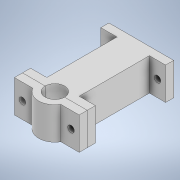
# Autodesk Inventor part: Держатель лазера
Saved by Autodesk Inventor 2022 (Build 260153000, 153)
## iProperties
Created: 2022-06-19
Part Number: Держатель лазера
Material: Типовые
Document SubType Name: Modeling
Designer: Admin
Density: 1 g/cm^3
Appearance: По умолчанию
Author: Admin
Autodesk Inventor part; units mm, degrees
ref_plane "YZ Plane" through (0, 0, 0) normal (1, 0, 0) x (0, 1, 0)
ref_plane "XZ Plane" through (0, 0, 0) normal (0, 1, 0) x (-1, 0, 0)
ref_plane "XY Plane" through (0, 0, 0) normal (0, 0, 1) x (1, 0, 0)
sketch "Эскиз1" plane through (0, 0, 0) normal (0, 0, 1) x (1, 0, 0)
  line L0 (20, -10) -> (-20, -10)
  line L1 (-20, -10) -> (-20, 10)
  line L2 (-20, 10) -> (20, 10)
  line L3 (20, 10) -> (20, -10)
  line L4 (20, -10) -> (-20, 10) construction
  line L5 (-20, -10) -> (20, 10) construction
  circle A0 centre (-15, 0) radius 2
  circle A1 centre (15, 0) radius 2
  line L6 (-10, -10) -> (10, -10)
  line L7 (10, -10) -> (10, 10)
  line L8 (10, 10) -> (-10, 10)
  line L9 (-10, 10) -> (-10, -10)
  line L10 (-10, -10) -> (10, 10) construction
  line L11 (10, -10) -> (-10, 10) construction
  point P0 (0, 0)
  point P1 (0, 0)
  dimension "d0" = 40
  dimension "d1" = 20
  dimension "d2" = 4
  dimension "d3" = 4
  dimension "d4" = 15
  dimension "d5" = 15
  dimension "d6" = 20
  constraints: 24 end point, 5 midpoint, 4 parallel, 2 centre point, 2 horizontal, 2 horizontal alignment, 2 perpendicular, 1 point on line
  measures "d0" distance of L1.end L2.end
  measures "d1" distance of L2.end L0.start
  measures "d2" diameter of A0
  measures "d3" diameter of A1
  measures "d4" distance of point (0, 0) A1.centre
  measures "d5" distance of point (0, 0) A0.centre
  measures "d6" distance between parallel lines of L9 L7
extrude "Выдавливание1" add sketch "Эскиз1" against normal blind 5 contours L0 L7 L2 L3 | L0 L9 L2 L7 | L0 L1 L2 L9 | A0 | A1
extrude "Выдавливание2" cut sketch "Эскиз1" against normal through all contours A0 | A1
extrude "Выдавливание3" add sketch "Эскиз1" along normal blind 48.359 contours L0 L9 L2 L7
sketch "Эскиз2" plane through (-20, -10, -5) normal (0, -1, 0) x (1, 0, 0)
  line L0 (30, 53.359) -> (10, 53.359) projected
  circle A0 centre (20, 53.359) radius 6
  point P0 (20, 5)
  dimension "d13" = 12
  constraints: 1 centre point, 1 midpoint
  measures "d13" diameter of A0
extrude "Выдавливание4" cut sketch "Эскиз2" against normal through all
sketch "Эскиз3" plane through (0, 0, 48.359) normal (0, 0, 1) x (1, 0, 0)
  line L0 (-20, 10) -> (20, 10) projected
  line L1 (-20, -10) -> (20, -10)
  line L2 (20, -10) -> (20, 10)
  line L3 (20, 10) -> (-20, 10)
  line L4 (-20, 10) -> (-20, -10)
  line L5 (-20, -10) -> (20, 10) construction
  line L6 (20, -10) -> (-20, 10) construction
  line L7 (-6, -10) -> (-6, 10) projected
  line L8 (6, 10) -> (6, -10) projected
  circle A0 centre (-15, 0) radius 2 projected
  circle A1 centre (15, 0) radius 2 projected
  point P0 (0, 0)
  constraints: 12 end point, 2 midpoint, 2 parallel, 1 horizontal, 1 perpendicular
extrude "Выдавливание5" add sketch "Эскиз3" against normal blind 5 contours L0 L7 L1 L4 | L0 L2 L1 L8
sketch "Эскиз4" plane through (-20, -10, -5) normal (0, -1, 0) x (1, 0, 0)
  circle A0 centre (20, 53.359) radius 6
  arc A1 (14, 53.359) -> (26, 53.359) centre (20, 53.359) ccw projected
  circle A2 centre (20, 53.359) radius 10
  line L0 (0, 53.359) -> (14, 53.359) projected
  line L1 (26, 53.359) -> (40, 53.359) projected
  line L2 (14, 53.359) -> (0, 53.359) projected
  line L3 (0, 53.359) -> (40, 53.359)
  line L4 (40, 53.359) -> (40, 58.359)
  line L5 (40, 58.359) -> (0, 58.359)
  line L6 (0, 58.359) -> (0, 53.359)
  point P0 (20, 5)
  point P1 (14, 53.359)
  point P2 (26, 53.359)
  point P3 (28.6603, 58.359)
  point P4 (11.3397, 58.359)
  dimension "d18" = 12
  dimension "d19" = 20
  dimension "d20" = 5
  constraints: 8 end point, 2 centre point, 2 coincident, 2 parallel, 1 concentric, 1 horizontal, 1 perpendicular
  measures "d18" diameter of A0
  measures "d19" diameter of A2
  measures "d20" distance of L4.end L3.end
extrude "Выдавливание6" add sketch "Эскиз4" against normal up to surface (20 mm away) separate body contours L0 A2 L5 A0 | A0 L5 A2 L1 | L5 A2 A0 | L0 L6 L5 A2 | A2 L5 L4 L1
extrude "Выдавливание7" cut sketch "Эскиз3" along normal through all contours A0 | A1 bodies 1 2
sketch "Эскиз5" plane through (0, 0, 43.359) normal (0, 0, -1) x (-1, 0, 0)
  line L0 (-11.5359, 0) -> (-13.2679, -3)
  line L1 (-13.2679, -3) -> (-16.7321, -3)
  line L2 (-16.7321, -3) -> (-18.4641, 0)
  line L3 (-18.4641, 0) -> (-16.7321, 3)
  line L4 (-16.7321, 3) -> (-13.2679, 3)
  line L5 (-13.2679, 3) -> (-11.5359, 0)
  line L6 (18.4641, 0) -> (16.7321, -3)
  line L7 (16.7321, -3) -> (13.2679, -3)
  line L8 (13.2679, -3) -> (11.5359, 0)
  line L9 (11.5359, 0) -> (13.2679, 3)
  line L10 (13.2679, 3) -> (16.7321, 3)
  line L11 (16.7321, 3) -> (18.4641, 0)
  circle A0 centre (15, 0) radius 2 projected
  circle A1 centre (-15, 0) radius 2 projected
  point P0 (0, 0)
  dimension "d25" = 6
  dimension "d26" = 6
  constraints: 24 end point, 4 horizontal alignment, 2 coincident, 26 other
  measures "d25" distance between parallel lines of L10 L7
  measures "d26" distance between parallel lines of L4 L1
extrude "Выдавливание8" cut sketch "Эскиз5" against normal blind 1 bodies 1
